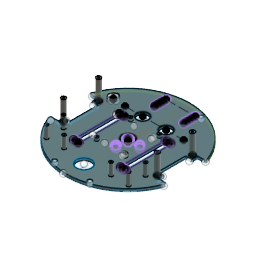
FEKTBOT_RPI_3or4_ver_1_2 (Autodesk Fusion 360 design; units mm, degrees)
Autodesk Fusion 360 part; units mm, degrees
note: some values were not read from the file. Set by a fixed rule: which sketch regions a step uses.
sketch "podklad" plane through (0, 0, 0) normal (0, 1, 0) x (1, 0, 0)
  line L0 (-75.0372, -23.4927) -> (-85, -23.4927)
  arc A0 (96.7123, 33.4364) -> (98.5902, 36.1245) centre (96.7123, 35.4364) ccw
  line L1 (85, -33.4277) -> (85, -23.4927)
  line L2 (-75.0372, -23.4927) -> (-75.0372, 23.5073)
  line L3 (74.9628, -23.4927) -> (74.9628, 23.5073)
  line L4 (0, 105) -> (0, -105) construction
  line L5 (-85, 23.5073) -> (-75.0372, 23.5073)
  arc A1 (-98.5902, 36.1245) -> (-96.7123, 33.4364) centre (-96.7123, 35.4364) ccw
  arc A2 (-96.7154, -33.4277) -> (-98.5934, -36.1156) centre (-96.7154, -35.4277) ccw
  line L6 (74.9628, -23.4927) -> (85, -23.4927)
  line L7 (85, 23.5073) -> (74.9628, 23.5073)
  line L8 (-85, 33.4364) -> (-85, 23.5073)
  arc A3 (-98.5934, -36.1156) -> (98.5934, -36.1156) centre (0, 0) ccw
  line L9 (85, 33.4364) -> (85, 23.5073)
  line L10 (96.7123, 33.4364) -> (85, 33.4364)
  line L11 (-96.7154, -33.4277) -> (-85, -33.4277)
  arc A4 (98.5934, -36.1156) -> (96.7154, -33.4277) centre (96.7154, -35.4277) ccw
  arc A5 (98.5902, 36.1245) -> (15, 103.923) centre (0, 0) ccw
  arc A6 (15, 103.923) -> (-15, 103.923) centre (0, 0) ccw
  arc A7 (-15, 103.923) -> (-98.5902, 36.1245) centre (0, 0) ccw
  line L12 (-96.7123, 33.4364) -> (-85, 33.4364)
  line L13 (96.7154, -33.4277) -> (85, -33.4277)
  line L14 (-85, -33.4277) -> (-85, -23.4927)
  circle A8 centre (30, -94.9953) radius 2.05
  line L15 (2.5, 0) -> (20, 0)
  line L16 (0, -20) -> (0, -2.5)
  circle A9 centre (-30, -94.9953) radius 2.05
  circle A10 centre (-30, 94.9953) radius 2.05
  circle A11 centre (30, 94.9953) radius 2.05
  line L17 (-79.8375, 50) -> (-70.1625, 50) construction
  line L18 (-75, 54.4496) -> (-75, 45.5504) construction
  line L19 (-77, 57.9) -> (-73, 57.9)
  line L20 (-73, 42.1) -> (-77, 42.1)
  line L21 (-73, 57.9) -> (-73, 56.9687)
  line L22 (-73, 43.0313) -> (-73, 42.1)
  line L23 (-77, 42.1) -> (-77, 43.0313)
  line L24 (-77, 56.9687) -> (-77, 57.9)
  arc A12 (-77, 56.9687) -> (-77, 43.0313) centre (-75, 50) ccw
  arc A13 (-73, 43.0313) -> (-73, 56.9687) centre (-75, 50) ccw
  point P0 (-7.5, -102.9967)
  point P1 (-82.0372, 22.8073)
  point P2 (-17.0372, -22.7927)
  point P3 (81.9628, 22.8073)
  point P4 (-0.0372, 0.0073)
  point P5 (-82.0372, -22.7927)
  point P6 (16.9628, 27.0073)
  point P7 (16.9628, 22.8073)
  point P8 (-17.0372, 27.0073)
  point P9 (16.9628, -22.7927)
  point P10 (81.9628, -22.7927)
  point P11 (16.9628, -26.9927)
  dimension "d1" = 210
  dimension "d2" = 2
  dimension "d3" = 2
  dimension "d4" = 2
  dimension "d5" = 2
  dimension "d39" = 4.1
  dimension "d215" = 14.5
  dimension "d216" = 15.8
  dimension "d217" = 4
  dimension "d218" = 50
  dimension "d219" = 75
  constraint horizontal L5
  constraint horizontal L0
  constraint horizontal L7
  constraint horizontal L6
  constraint horizontal L12
  constraint vertical L8
  constraint horizontal L11
  constraint vertical L14
  constraint horizontal L13
  constraint vertical L1
  constraint horizontal L10
  constraint vertical L9
  constraint coincident A3.centre A5.centre
  constraint tangent A2 A3
  constraint tangent A2 L11
  constraint tangent A1 A5
  constraint tangent A1 L12
  constraint tangent A0 L10
  constraint tangent A0 A5
  constraint tangent A4 L13
  constraint tangent A3 A4
  constraint midpoint L4.end A3
  constraint concentric A5 A7
  constraint coincident L4.start A5
  constraint vertical L3
  constraint vertical L2
  constraint coincident L4.start A6
  constraint symmetric A8 L16 A9
  constraint symmetric A8 L15 A11
  constraint symmetric L15 A9 A10
  constraint horizontal L17
  constraint perpendicular L17 L18
  constraint midpoint L18 A12.centre
  constraint horizontal L19
  constraint vertical L21
  constraint horizontal L20
  constraint vertical L23
  constraint symmetric L18 L22 L23
  constraint symmetric L17 L19 L20
  constraint midpoint L17 A12.centre
  constraint collinear L21 L22
  constraint collinear L23 L24
  constraint concentric A12 A13
  measures "d1" diameter of A5 L4
  measures "d2" radius of A2
  measures "d3" radius of A1
  measures "d4" radius of A0
  measures "d5" radius of A4
  measures "d39" diameter of A8
  measures "d57" diameter of L0.end
  measures "d215" diameter of A12
  measures "d216" distance of L19.start L20.end
  measures "d217" distance of L19.start L19.end
  measures "d218" distance of L15 L17
  measures "d219" distance of L16 L18
extrude "Extrude1" add sketch "podklad" along normal blind 4 contours L0 A0 L1 L2 L3 L5 A1 A2 L6 L7 L8 A3 L9 L10 L11 A4 A5 A6 A7 L12 L13 L14 | A9 | A10 | A11 | L19 L20 L21 L22 L23 L24 A12 A13
sketch "diry_hlavy_sroubu" plane through (0, 4, 0) normal (0, 1, 0) x (-1, 0, 0)
  circle A0 centre (-30, 94.9953) radius 2.05
  arc A1 (96.7154, 33.4277) -> (98.5934, 36.1156) centre (96.7154, 35.4277) ccw
  arc A2 (98.5934, 36.1156) -> (-98.5934, 36.1156) centre (0, 0) ccw
  arc A3 (-98.5934, 36.1156) -> (-96.7154, 33.4277) centre (-96.7154, 35.4277) ccw
  line L0 (-96.7154, 33.4277) -> (-85, 33.4277)
  line L1 (-85, 33.4277) -> (-85, 23.4927)
  line L2 (-85, 23.4927) -> (-74.9628, 23.4927)
  line L3 (-74.9628, 23.4927) -> (-74.9628, -23.5073)
  line L4 (-74.9628, -23.5073) -> (-85, -23.5073)
  line L5 (-85, -23.5073) -> (-85, -33.4364)
  line L6 (-85, -33.4364) -> (-96.7123, -33.4364)
  arc A4 (-96.7123, -33.4364) -> (-98.5902, -36.1245) centre (-96.7123, -35.4364) ccw
  arc A5 (-98.5902, -36.1245) -> (98.5902, -36.1245) centre (0, 0) ccw
  arc A6 (98.5902, -36.1245) -> (96.7123, -33.4364) centre (96.7123, -35.4364) ccw
  line L7 (96.7123, -33.4364) -> (85, -33.4364)
  line L8 (85, -33.4364) -> (85, -23.5073)
  line L9 (85, -23.5073) -> (75.0372, -23.5073)
  line L10 (75.0372, -23.5073) -> (75.0372, 23.4927)
  line L11 (75.0372, 23.4927) -> (85, 23.4927)
  line L12 (85, 23.4927) -> (85, 33.4277)
  line L13 (85, 33.4277) -> (96.7154, 33.4277)
  circle A7 centre (29.9934, -95.0047) radius 3.5
  circle A8 centre (-29.9934, -95.0047) radius 3.5
  circle A9 centre (30, 94.9953) radius 3.5
  circle A10 centre (-30, 94.9953) radius 3.5
  dimension "d55" = 7
  dimension "d56" = 7
  dimension "d57" = 7
  dimension "d58" = 7
  constraint concentric A0 A10
  measures "d55" diameter of A7
  measures "d56" diameter of A8
  measures "d57" diameter of A9
  measures "d58" diameter of A10
extrude "Extrude3" cut sketch "diry_hlavy_sroubu" against normal blind 3 contours A7 | A8 | A9 | A10
sketch "sloupky_rpi" plane through (0, 4, 0) normal (0, 1, 0) x (-1, 0, 0)
  circle A0 centre (-30, 94.9953) radius 3.5
  circle A1 centre (29.9934, -95.0047) radius 3.5
  circle A2 centre (30, 94.9953) radius 3.5
  circle A3 centre (-29.9934, -95.0047) radius 3.5
  arc A4 (96.7154, 33.4277) -> (98.5934, 36.1156) centre (96.7154, 35.4277) ccw
  arc A5 (98.5934, 36.1156) -> (-98.5934, 36.1156) centre (0, 0) ccw
  arc A6 (-98.5934, 36.1156) -> (-96.7154, 33.4277) centre (-96.7154, 35.4277) ccw
  line L0 (-96.7154, 33.4277) -> (-85, 33.4277)
  line L1 (-85, 33.4277) -> (-85, 23.4927)
  line L2 (-85, 23.4927) -> (-74.9628, 23.4927)
  line L3 (-74.9628, 23.4927) -> (-74.9628, -23.5073)
  line L4 (-74.9628, -23.5073) -> (-85, -23.5073)
  line L5 (-85, -23.5073) -> (-85, -33.4364)
  line L6 (-85, -33.4364) -> (-96.7123, -33.4364)
  arc A7 (-96.7123, -33.4364) -> (-98.5902, -36.1245) centre (-96.7123, -35.4364) ccw
  arc A8 (-98.5902, -36.1245) -> (98.5902, -36.1245) centre (0, 0) ccw
  arc A9 (98.5902, -36.1245) -> (96.7123, -33.4364) centre (96.7123, -35.4364) ccw
  line L7 (96.7123, -33.4364) -> (85, -33.4364)
  line L8 (85, -33.4364) -> (85, -23.5073)
  line L9 (85, -23.5073) -> (75.0372, -23.5073)
  line L10 (75.0372, -23.5073) -> (75.0372, 23.4927)
  line L11 (75.0372, 23.4927) -> (85, 23.4927)
  line L12 (85, 23.4927) -> (85, 33.4277)
  line L13 (85, 33.4277) -> (96.7154, 33.4277)
  line L14 (24.5, -29) -> (-24.5, -29) construction
  line L15 (-24.5, -29) -> (-24.5, 29) construction
  line L16 (-24.5, 29) -> (24.5, 29) construction
  line L17 (24.5, 29) -> (24.5, -29) construction
  line L18 (0, 1.75) -> (0, 22.5)
  line L19 (-2.5, 0) -> (-20, 0)
  circle A10 centre (-24.5, -29) radius 1.2
  circle A11 centre (-24.5, -29) radius 3
  circle A12 centre (24.5, -29) radius 1.2
  circle A13 centre (24.5, -29) radius 3
  circle A14 centre (24.5, 29) radius 1.2
  circle A15 centre (24.5, 29) radius 3
  circle A16 centre (-24.5, 29) radius 1.2
  circle A17 centre (-24.5, 29) radius 3
  dimension "d159" = 49
  dimension "d160" = 58
  dimension "d161" = 29
  dimension "d162" = 2.4
  dimension "d163" = 6
  dimension "d164" = 2.4
  dimension "d165" = 6
  dimension "d166" = 2.4
  dimension "d167" = 6
  dimension "d168" = 2.4
  dimension "d169" = 6
  constraint horizontal L14
  constraint vertical L15
  constraint horizontal L16
  constraint vertical L17
  constraint symmetric L15 L17 L18
  constraint coincident L14.end L15.start
  constraint concentric A10 A11
  constraint coincident L14.start L17.end
  constraint concentric A12 A13
  constraint coincident L16.end L17.start
  constraint concentric A14 A15
  constraint coincident L15.end L16.start
  constraint concentric A16 A17
  measures "d159" distance of L14.start L14.end
  measures "d160" distance of L14.start L16.end
  measures "d161" distance of L14 L19
  measures "d162" diameter of A10
  measures "d163" diameter of A11
  measures "d164" diameter of A12
  measures "d165" diameter of A13
  measures "d166" diameter of A14
  measures "d167" diameter of A15
  measures "d168" diameter of A16
  measures "d169" diameter of A17
extrude "Extrude19" add sketch "sloupky_rpi" along normal blind 5 contours A11 | A13 | A15 | A17
extrude "Extrude20" cut 4 faces at (-23.7873, 4, 29.3432) (25.0231, 4, 28.6755) (25.2559, 4, -28.7668) (-23.7873, 4, -28.6568) along direction (0, -1, 0) blind 3
sketch "pruchodky" plane through (0, 4, 0) normal (0, 1, 0) x (-1, 0, 0)
  circle A0 centre (24.5, 29) radius 3
  circle A1 centre (24.5, -29) radius 3
  circle A2 centre (-30, 94.9953) radius 3.5
  circle A3 centre (29.9934, -95.0047) radius 3.5
  circle A4 centre (30, 94.9953) radius 3.5
  circle A5 centre (-29.9934, -95.0047) radius 3.5
  arc A6 (96.7154, 33.4277) -> (98.5934, 36.1156) centre (96.7154, 35.4277) ccw
  arc A7 (98.5934, 36.1156) -> (-98.5934, 36.1156) centre (0, 0) ccw
  arc A8 (-98.5934, 36.1156) -> (-96.7154, 33.4277) centre (-96.7154, 35.4277) ccw
  line L0 (-96.7154, 33.4277) -> (-85, 33.4277)
  line L1 (-85, 33.4277) -> (-85, 23.4927)
  line L2 (-85, 23.4927) -> (-74.9628, 23.4927)
  line L3 (-74.9628, 23.4927) -> (-74.9628, -23.5073)
  line L4 (-74.9628, -23.5073) -> (-85, -23.5073)
  line L5 (-85, -23.5073) -> (-85, -33.4364)
  line L6 (-85, -33.4364) -> (-96.7123, -33.4364)
  arc A9 (-96.7123, -33.4364) -> (-98.5902, -36.1245) centre (-96.7123, -35.4364) ccw
  arc A10 (-98.5902, -36.1245) -> (98.5902, -36.1245) centre (0, 0) ccw
  arc A11 (98.5902, -36.1245) -> (96.7123, -33.4364) centre (96.7123, -35.4364) ccw
  line L7 (96.7123, -33.4364) -> (85, -33.4364)
  line L8 (85, -33.4364) -> (85, -23.5073)
  line L9 (85, -23.5073) -> (75.0372, -23.5073)
  line L10 (75.0372, -23.5073) -> (75.0372, 23.4927)
  line L11 (75.0372, 23.4927) -> (85, 23.4927)
  line L12 (85, 23.4927) -> (85, 33.4277)
  line L13 (85, 33.4277) -> (96.7154, 33.4277)
  circle A12 centre (-24.5, -29) radius 3
  circle A13 centre (-24.5, 29) radius 3
  line L14 (25, -90) -> (-25, -90) construction
  line L15 (0, 1.75) -> (0, 22.5) construction
  line L16 (-2.5, 0) -> (-20, 0) construction
  circle A14 centre (25, -90) radius 1.55
  circle A15 centre (-25, -90) radius 1.5
  circle A16 centre (0, 0) radius 10
  line L17 (50, -45) -> (-50, -45) construction
  circle A17 centre (50, -45) radius 3.5
  circle A18 centre (-50, -45) radius 3.5
  circle A19 centre (20, -45) radius 9.6
  circle A20 centre (-20, -45) radius 9.6
  line L18 (0, 20) -> (0, 2.5)
  circle A21 centre (0.0755, 75) radius 12.5
  line L19 (37, -30) -> (43, -30)
  line L20 (45, -28) -> (45, 48)
  line L21 (43, 50) -> (37, 50)
  line L22 (35, 48) -> (35, -28)
  arc A22 (43, -30) -> (45, -28) centre (43, -28) ccw
  arc A23 (35, -28) -> (37, -30) centre (37, -28) ccw
  arc A24 (45, 48) -> (43, 50) centre (43, 48) ccw
  arc A25 (37, 50) -> (35, 48) centre (37, 48) ccw
  line L23 (-45, -28) -> (-45, 48)
  line L24 (-37, -30) -> (-43, -30)
  line L25 (-35, 48) -> (-35, -28)
  line L26 (-43, 50) -> (-37, 50)
  arc A26 (-45, -28) -> (-43, -30) centre (-43, -28) ccw
  arc A27 (-37, -30) -> (-35, -28) centre (-37, -28) ccw
  arc A28 (-43, 50) -> (-45, 48) centre (-43, 48) ccw
  arc A29 (-35, 48) -> (-37, 50) centre (-37, 48) ccw
  circle A30 centre (-25, -85) radius 1.5
  circle A31 centre (25, -85) radius 1.55
  circle A32 centre (-25, -80) radius 1.5
  circle A33 centre (25, -80) radius 1.55
  circle A34 centre (-25, -75) radius 1.5
  circle A35 centre (25, -75) radius 1.55
  circle A36 centre (-25, -70) radius 1.5
  circle A37 centre (25, -70) radius 1.55
  point P0 (45, -25)
  point P1 (35, 25)
  point P2 (35, -30)
  point P3 (45, -30)
  point P4 (35, 50)
  point P5 (25, -85)
  point P6 (25, -80)
  point P7 (25, -75)
  point P8 (25, -70)
  dimension "d174" = 50
  dimension "d175" = 90
  dimension "d176" = 3.1
  dimension "d177" = 3
  dimension "d178" = 20
  dimension "d187" = 100
  dimension "d188" = 45
  dimension "d189" = 7
  dimension "d190" = 7
  dimension "d191" = 19.2
  dimension "d192" = 19.2
  dimension "d193" = 30
  dimension "d194" = 30
  dimension "d199" = 25
  dimension "d200" = 75
  dimension "d210" = 10
  dimension "d211" = 80
  dimension "d212" = 35
  dimension "d213" = 30
  dimension "d214" = 2
  dimension "d222" = 0
  dimension "d223" = 5
  constraint horizontal L14
  constraint symmetric L14.start L14.end L15
  constraint coincident L14.start A14.centre
  constraint coincident L14.end A15.centre
  constraint concentric A7 A16
  constraint horizontal L17
  constraint symmetric L15 L17.start L17.end
  constraint coincident L17.start A17.centre
  constraint coincident L17.end A18.centre
  constraint coincident L17 A19.centre
  constraint coincident L17 A20.centre
  constraint horizontal L19
  constraint vertical L20
  constraint horizontal L21
  constraint vertical L22
  constraint coincident P3 L19
  constraint coincident P3 L20
  constraint tangent L19 A22
  constraint tangent L20 A22
  constraint coincident P2 L19
  constraint coincident P2 L22
  constraint tangent L19 A23
  constraint tangent L22 A23
  constraint equal A22 A23
  constraint tangent L20 A24
  constraint tangent L21 A24
  constraint equal A22 A24
  constraint coincident P4 L21
  constraint coincident P4 L22
  constraint tangent L21 A25
  constraint tangent L22 A25
  constraint equal A22 A25
  constraint symmetric L18 L19.end L24.end
  constraint symmetric L18 L20.start L23.start
  constraint symmetric L18 A22 A26
  constraint symmetric L18 L19.start L24.start
  constraint symmetric L18 L22.end L25.end
  constraint symmetric L18 A23 A27
  constraint symmetric L18 L20.end L23.end
  constraint symmetric L18 L21.start L26.start
  constraint symmetric L18 A24 A28
  constraint symmetric L18 L21.end L26.end
  constraint symmetric L18 L22.start L25.start
  constraint symmetric L18 A25 A29
  measures "d174" distance of L14.start L14.end
  measures "d175" distance of L14 L16
  measures "d176" diameter of A14
  measures "d177" diameter of A15
  measures "d178" diameter of A16
  measures "d187" distance of L17.start L17.end
  measures "d188" distance of L16 L17
  measures "d189" diameter of A17
  measures "d190" diameter of A18
  measures "d191" diameter of A19
  measures "d192" diameter of A20
  measures "d193" distance of L17.start A19.centre
  measures "d194" distance of L17.end A20.centre
  measures "d199" diameter of A21
  measures "d200" distance of L16 A21.centre
  measures "d210" distance of P2 P3
  measures "d211" distance of P2 P4
  measures "d212" distance of L18 L22
  measures "d213" distance of L16 L19
  measures "d214" radius of A22
extrude "Extrude22" cut sketch "pruchodky" against normal blind 10 contours A14 | A15 | A16 | A17 | A18 | A19 | A20 | A21 | L19 L20 L21 L22 A22 A23 A24 A25 | L23 L24 L25 L26 A26 A27 A28 A29 | A30 | A31 | A32 | A33 | A34 | A35 | A36 | A37
sketch "dalsi_patro" plane through (0, 4, 0) normal (0, 1, 0) x (-1, 0, 0)
  circle A0 centre (24.5, 29) radius 3
  circle A1 centre (24.5, -29) radius 3
  circle A2 centre (-30, 94.9953) radius 3.5
  circle A3 centre (29.9934, -95.0047) radius 3.5
  circle A4 centre (30, 94.9953) radius 3.5
  circle A5 centre (-29.9934, -95.0047) radius 3.5
  arc A6 (96.7154, 33.4277) -> (98.5934, 36.1156) centre (96.7154, 35.4277) ccw
  arc A7 (98.5934, 36.1156) -> (-98.5934, 36.1156) centre (0, 0) ccw
  arc A8 (-98.5934, 36.1156) -> (-96.7154, 33.4277) centre (-96.7154, 35.4277) ccw
  line L0 (-96.7154, 33.4277) -> (-85, 33.4277)
  line L1 (-85, 33.4277) -> (-85, 23.4927)
  line L2 (-85, 23.4927) -> (-74.9628, 23.4927)
  line L3 (-74.9628, 23.4927) -> (-74.9628, -23.5073)
  line L4 (-74.9628, -23.5073) -> (-85, -23.5073)
  line L5 (-85, -23.5073) -> (-85, -33.4364)
  line L6 (-85, -33.4364) -> (-96.7123, -33.4364)
  arc A9 (-96.7123, -33.4364) -> (-98.5902, -36.1245) centre (-96.7123, -35.4364) ccw
  arc A10 (-98.5902, -36.1245) -> (98.5902, -36.1245) centre (0, 0) ccw
  arc A11 (98.5902, -36.1245) -> (96.7123, -33.4364) centre (96.7123, -35.4364) ccw
  line L7 (96.7123, -33.4364) -> (85, -33.4364)
  line L8 (85, -33.4364) -> (85, -23.5073)
  line L9 (85, -23.5073) -> (75.0372, -23.5073)
  line L10 (75.0372, -23.5073) -> (75.0372, 23.4927)
  line L11 (75.0372, 23.4927) -> (85, 23.4927)
  line L12 (85, 23.4927) -> (85, 33.4277)
  line L13 (85, 33.4277) -> (96.7154, 33.4277)
  circle A12 centre (-24.5, -29) radius 3
  circle A13 centre (-24.5, 29) radius 3
  circle A14 centre (0, 0) radius 10
  circle A15 centre (50, -45) radius 3.5
  circle A16 centre (20, -45) radius 9.6
  circle A17 centre (0.0755, 75) radius 12.5
  circle A18 centre (-50, -45) radius 3.5
  circle A19 centre (-20, -45) radius 9.6
  circle A20 centre (80, 30) radius 4
  line L14 (0, 20) -> (0, 2.5)
  line L15 (-2.5, 0) -> (-20, 0)
  circle A21 centre (80, 30) radius 1.45
  circle A22 centre (-80, 30) radius 4
  circle A23 centre (-80, 30) radius 1.45
  circle A24 centre (80, -30) radius 4
  circle A25 centre (-80, -30) radius 4
  circle A26 centre (-80, -30) radius 1.45
  circle A27 centre (80, -30) radius 1.45
  line L16 (-35, 48) -> (-35, -28)
  arc A28 (-37, -30) -> (-35, -28) centre (-37, -28) ccw
  line L17 (-37, -30) -> (-43, -30)
  arc A29 (-45, -28) -> (-43, -30) centre (-43, -28) ccw
  line L18 (-45, -28) -> (-45, 48)
  arc A30 (-43, 50) -> (-45, 48) centre (-43, 48) ccw
  line L19 (-43, 50) -> (-37, 50)
  arc A31 (-35, 48) -> (-37, 50) centre (-37, 48) ccw
  line L20 (35, -28) -> (35, 48)
  arc A32 (37, 50) -> (35, 48) centre (37, 48) ccw
  line L21 (37, 50) -> (43, 50)
  arc A33 (45, 48) -> (43, 50) centre (43, 48) ccw
  line L22 (45, 48) -> (45, -28)
  arc A34 (43, -30) -> (45, -28) centre (43, -28) ccw
  line L23 (43, -30) -> (37, -30)
  arc A35 (35, -28) -> (37, -30) centre (37, -28) ccw
  circle A36 centre (-25, -90) radius 1.5
  circle A37 centre (25, -90) radius 1.55
  circle A38 centre (-25, -70) radius 1.5
  circle A39 centre (25, -85) radius 1.55
  circle A40 centre (25, -70) radius 1.55
  circle A41 centre (-25, -85) radius 1.5
  circle A42 centre (-25, -75) radius 1.5
  circle A43 centre (25, -80) radius 1.55
  circle A44 centre (25, -75) radius 1.55
  circle A45 centre (-25, -80) radius 1.5
  dimension "d203" = 8
  dimension "d204" = 80
  dimension "d205" = 30
  dimension "d206" = 2.9
  constraint concentric A20 A21
  constraint symmetric A20 L14 A22
  constraint symmetric L14 A21 A23
  constraint symmetric A20 L15 A24
  constraint symmetric L15 A21 A27
  constraint symmetric L15 A22 A25
  constraint symmetric L15 A23 A26
  measures "d203" diameter of A20
  measures "d204" distance of A20.centre L14
  measures "d205" distance of A20.centre L15
  measures "d206" diameter of A21
extrude "Extrude23" add sketch "dalsi_patro" along normal blind 35 contours A20 | A22 | A24 | A25
extrude "Extrude24" cut sketch "podklad" along normal blind 10 contours A9 | A10 | A11 | L19 L20 L21 L22 L23 L24 A12 A13
sketch "oled_sloupky" plane through (0, 4, 0) normal (0, 1, 0) x (-1, 0, 0)
  circle A0 centre (-80, -30) radius 4
  circle A1 centre (-80, 30) radius 4
  circle A2 centre (-25, -80) radius 1.5
  circle A3 centre (25, -75) radius 1.55
  line L0 (-35, 48) -> (-35, -28)
  arc A4 (-37, -30) -> (-35, -28) centre (-37, -28) ccw
  line L1 (-37, -30) -> (-43, -30)
  arc A5 (-45, -28) -> (-43, -30) centre (-43, -28) ccw
  line L2 (-45, -28) -> (-45, 48)
  arc A6 (-43, 50) -> (-45, 48) centre (-43, 48) ccw
  line L3 (-43, 50) -> (-37, 50)
  arc A7 (-35, 48) -> (-37, 50) centre (-37, 48) ccw
  circle A8 centre (50, -45) radius 3.5
  circle A9 centre (20, -45) radius 9.6
  circle A10 centre (0.0755, 75) radius 12.5
  circle A11 centre (25, -90) radius 1.55
  circle A12 centre (25, -80) radius 1.55
  circle A13 centre (-25, -75) radius 1.5
  circle A14 centre (-25, -85) radius 1.5
  circle A15 centre (25, -70) radius 1.55
  line L4 (35, -28) -> (35, 48)
  arc A16 (37, 50) -> (35, 48) centre (37, 48) ccw
  line L5 (37, 50) -> (43, 50)
  arc A17 (45, 48) -> (43, 50) centre (43, 48) ccw
  line L6 (45, 48) -> (45, -28)
  arc A18 (43, -30) -> (45, -28) centre (43, -28) ccw
  line L7 (43, -30) -> (37, -30)
  arc A19 (35, -28) -> (37, -30) centre (37, -28) ccw
  circle A20 centre (-50, -45) radius 3.5
  circle A21 centre (-20, -45) radius 9.6
  circle A22 centre (0, 0) radius 10
  circle A23 centre (-25, -90) radius 1.5
  circle A24 centre (25, -85) radius 1.55
  circle A25 centre (-25, -70) radius 1.5
  circle A26 centre (24.5, 29) radius 3
  circle A27 centre (24.5, -29) radius 3
  circle A28 centre (-30, 94.9953) radius 3.5
  circle A29 centre (29.9934, -95.0047) radius 3.5
  circle A30 centre (30, 94.9953) radius 3.5
  circle A31 centre (-29.9934, -95.0047) radius 3.5
  arc A32 (96.7154, 33.4277) -> (98.5934, 36.1156) centre (96.7154, 35.4277) ccw
  arc A33 (98.5934, 36.1156) -> (-98.5934, 36.1156) centre (0, 0) ccw
  arc A34 (-98.5934, 36.1156) -> (-96.7154, 33.4277) centre (-96.7154, 35.4277) ccw
  line L8 (-96.7154, 33.4277) -> (-85, 33.4277)
  line L9 (-85, 33.4277) -> (-85, 23.4927)
  line L10 (-85, 23.4927) -> (-74.9628, 23.4927)
  line L11 (-74.9628, 23.4927) -> (-74.9628, -23.5073)
  line L12 (-74.9628, -23.5073) -> (-85, -23.5073)
  line L13 (-85, -23.5073) -> (-85, -33.4364)
  line L14 (-85, -33.4364) -> (-96.7123, -33.4364)
  arc A35 (-96.7123, -33.4364) -> (-98.5902, -36.1245) centre (-96.7123, -35.4364) ccw
  arc A36 (-98.5902, -36.1245) -> (98.5902, -36.1245) centre (0, 0) ccw
  arc A37 (98.5902, -36.1245) -> (96.7123, -33.4364) centre (96.7123, -35.4364) ccw
  line L15 (96.7123, -33.4364) -> (85, -33.4364)
  line L16 (85, -33.4364) -> (85, -23.5073)
  line L17 (85, -23.5073) -> (75.0372, -23.5073)
  line L18 (75.0372, -23.5073) -> (75.0372, 23.4927)
  line L19 (75.0372, 23.4927) -> (85, 23.4927)
  line L20 (85, 23.4927) -> (85, 33.4277)
  line L21 (85, 33.4277) -> (96.7154, 33.4277)
  circle A38 centre (-24.5, -29) radius 3
  circle A39 centre (-24.5, 29) radius 3
  circle A40 centre (80, 30) radius 4
  circle A41 centre (80, -30) radius 4
  line L22 (73, -42.1) -> (77, -42.1)
  line L23 (77, -42.1) -> (77, -43.0313)
  arc A42 (77, -56.9687) -> (77, -43.0313) centre (75, -50) ccw
  line L24 (77, -56.9687) -> (77, -57.9)
  line L25 (77, -57.9) -> (73, -57.9)
  line L26 (73, -57.9) -> (73, -56.9687)
  arc A43 (73, -43.0313) -> (73, -56.9687) centre (75, -50) ccw
  line L27 (73, -43.0313) -> (73, -42.1)
  line L28 (-70, 69) -> (-40, 69) construction
  line L29 (-40, 69) -> (-40, 40) construction
  line L30 (-40, 40) -> (-70, 40) construction
  line L31 (-70, 40) -> (-70, 69) construction
  line L32 (-2.5, 0) -> (-20, 0) construction
  line L33 (0, 20) -> (0, 2.5) construction
  circle A44 centre (-70, 69) radius 3
  circle A45 centre (-70, 40) radius 3
  circle A46 centre (-40, 69) radius 3
  circle A47 centre (-70, 69) radius 1.2
  circle A48 centre (-70, 40) radius 1.2
  circle A49 centre (-40, 69) radius 1.2
  circle A50 centre (40, 69) radius 3
  circle A51 centre (40, 69) radius 1.2
  circle A52 centre (70, 69) radius 3
  circle A53 centre (70, 69) radius 1.2
  circle A54 centre (70, 40) radius 3
  circle A55 centre (70, 40) radius 1.2
  dimension "d226" = 30
  dimension "d227" = 29
  dimension "d228" = 40
  dimension "d229" = 40
  dimension "d231" = 6
  dimension "d232" = 6
  dimension "d233" = 6
  dimension "d234" = 2.4
  dimension "d235" = 2.4
  dimension "d236" = 2.4
  constraint horizontal L28
  constraint vertical L29
  constraint horizontal L30
  constraint vertical L31
  constraint coincident L28.start L31.end
  constraint coincident L30.end L31.start
  constraint coincident L28.end L29.start
  constraint concentric A44 A47
  constraint concentric A45 A48
  constraint concentric A46 A49
  constraint symmetric L33 A44 A52
  constraint symmetric L33 A45 A54
  constraint symmetric L33 A46 A50
  constraint symmetric L33 A47 A53
  constraint symmetric L33 A48 A55
  constraint symmetric L33 A49 A51
  measures "d226" distance of L28.start L28.end
  measures "d227" distance of L28.start L30.end
  measures "d228" distance of L30 L32
  measures "d229" distance of L29 L33
  measures "d231" diameter of A44
  measures "d232" diameter of A45
  measures "d233" diameter of A46
  measures "d234" diameter of A47
  measures "d235" diameter of A48
  measures "d236" diameter of A49
extrude "Extrude25" add sketch "oled_sloupky" along normal blind 20 contours A44 | A45 | A46 | A50 | A52 | A54
equation "d161 = ( 58 / 2 ) * 1 mm"
